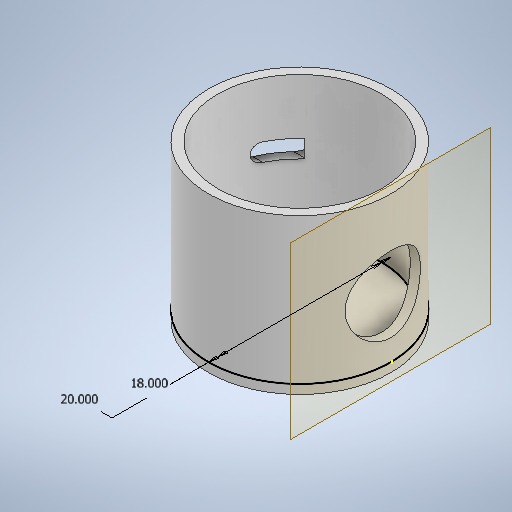
# Autodesk Inventor part: Part1
Saved by Autodesk Inventor 2025.1 (Build 291241020, 241B)
## iProperties
Created: 2024-10-30
Part Number: Part1
Material: Generic
Document SubType Name: Modeling
Designer: Krishnu
Density: 1 g/cm^3
Appearance: Default
Author: Krishnu
Autodesk Inventor part; units mm, degrees
ref_plane "XZ Plane" through (0, 0, 0) normal (0, 1, 0) x (-1, 0, 0)
ref_plane "XY Plane" through (0, 0, 0) normal (0, 0, 1) x (1, 0, 0)
sketch "Sketch1" plane through (0, 0, 0) normal (0, 1, 0) x (-1, 0, 0)
  circle A0 centre (0, 0) radius 228.6
  circle A1 centre (0, 0) radius 254
  dimension "d0" = 457.2
  dimension "d1" = 508
  constraints: 2 centre point, 2 coincident
  measures "d0" diameter of A0
  measures "d1" diameter of A1
extrude "Extrusion1" add sketch "Sketch1" along normal blind 406.4
sketch "Sketch2" plane through (0, 0, 0) normal (0, -1, 0) x (1, 0, 0)
  circle A0 centre (0, 0) radius 254
  constraints: 1 centre point, 1 coincident
extrude "Extrusion2" add sketch "Sketch2" along normal blind 25.4
ref_plane "Work Plane1" through (-254, 0, 0) normal (1, 0, 0) x (0, 1, 0)
sketch "Sketch3" plane through (-254, 0, 0) normal (1, 0, 0) x (0, 1, 0)
  line L0 (227.1973, -170.7692) -> (227.1973, -101.4716) construction
  line L1 (251.9465, -170.7692) -> (251.9465, -101.4716)
  line L2 (202.4481, -101.4716) -> (202.4481, -170.7692)
  arc A0 (202.4481, -170.7692) -> (251.9465, -170.7692) centre (227.1973, -170.7692) ccw
  arc A1 (251.9465, -101.4716) -> (202.4481, -101.4716) centre (227.1973, -101.4716) ccw
  point P0 (0, 0)
  point P1 (227.1973, -136.1204)
  constraints: 8 end point, 4 point on circle, 4 tangent, 2 centre point, 1 midpoint, 1 parallel, 1 vertical
extrude "Extrusion3" cut sketch "Sketch3" along normal blind 98.425
ref_plane "Plane for hole making" through (254, 0, 0) normal (1, 0, 0) x (0, 1, 0)
sketch "Sketch4" plane through (254, 0, 0) normal (1, 0, 0) x (0, 1, 0)
  point P0 (0, 0)
sketch "Sketch5" plane through (254, 0, 0) normal (1, 0, 0) x (0, 1, 0)
  circle A0 centre (164.2862, 0) radius 104.8554
  point P0 (0, 0)
  constraints: 1 centre point
extrude "Extrusion4" cut sketch "Sketch5" against normal blind 76.2
body "Solid1"
